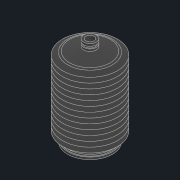
# Autodesk Inventor part: MCEN4000:T7
Saved by Autodesk Inventor 2021 (Build 250183000, 183)
## iProperties
Created: 2020-10-22
Part Number: MCEN4000:T7
Material: RUBBER, SILICONE
Document SubType Name: Modeling
Designer: Tang Kang Ning
Mass: 90.957 g
Surface Area: 1680.71 cm^2
Volume: 81.2116 cm^3
Density: 1.12 g/cm^3
Appearance: Rubber - Black
Description: BALL JOINT BELLOW
RevolveDIA: 7.056 mm
Author: Tang Kang Ning
Autodesk Inventor part; units mm, degrees
ref_plane "YZ Plane" through (0, 0, 0) normal (1, 0, 0) x (0, 1, 0)
ref_plane "XZ Plane" through (0, 0, 0) normal (0, 1, 0) x (-1, 0, 0)
ref_plane "XY Plane" through (0, 0, 0) normal (0, 0, 1) x (1, 0, 0)
sketch "Sketch1" plane through (0, 0, 0) normal (0, 0, 1) x (1, 0, 0)
  line L0 (-37, 65.25) -> (37, 65.25) projected
  line L1 (-37, 53.25) -> (37, 53.25) projected
  line L2 (35, 65.25) -> (35, 53.25)
  line L3 (7.056, 209) -> (7.056, 197)
  line L4 (7.056, 209) -> (7.056, 197)
  line L5 (9.056, 197) -> (7.056, 197)
  line L6 (7.056, 209) -> (11.056, 209)
  line L7 (35, 53.25) -> (39, 53.25)
  line L8 (39, 53.25) -> (39, 57.25)
  line L9 (39, 57.25) -> (37, 57.25)
  line L10 (37, 57.25) -> (37, 61.25)
  line L11 (37, 61.25) -> (39, 61.25)
  line L12 (39, 61.25) -> (39, 65.25)
  line L13 (39, 65.25) -> (37, 65.25) construction
  line L14 (11.056, 209) -> (11.056, 205)
  line L15 (11.056, 205) -> (9.056, 205)
  line L16 (9.056, 205) -> (9.056, 201)
  line L17 (9.056, 201) -> (11.056, 201)
  line L18 (11.056, 201) -> (11.056, 197)
  line L19 (39, 65.25) -> (47.9764, 69.6572)
  line L20 (37, 65.25) -> (45.9764, 69.6572)
  line L21 (37, 65.25) -> (37, 83.6946) construction
  line L22 (45.9764, 69.6572) -> (37, 69.6572) construction
  line L23 (45.9764, 69.6572) -> (37, 74.0645)
  line L24 (47.9764, 69.6572) -> (39, 74.0645)
  line L25 (35.5321, 190.0108) -> (11.056, 197.3225)
  line L26 (37, 188.6524) -> (9.056, 197)
  line L27 (37, 74.0645) -> (46.1526, 74.0645) construction
  line L28 (45.9764, 78.4717) -> (37, 82.8789)
  line L29 (47.9764, 78.4717) -> (39, 82.8789)
  line L30 (39, 74.0645) -> (47.9764, 78.4717)
  line L31 (37, 74.0645) -> (45.9764, 78.4717)
  line L32 (45.9764, 87.2861) -> (37, 91.6934)
  line L33 (47.9764, 87.2861) -> (39, 91.6934)
  line L34 (39, 82.8789) -> (47.9764, 87.2861)
  line L35 (37, 82.8789) -> (45.9764, 87.2861)
  line L36 (45.9764, 96.1006) -> (37, 100.5078)
  line L37 (47.9764, 96.1006) -> (39, 100.5078)
  line L38 (39, 91.6934) -> (47.9764, 96.1006)
  line L39 (37, 91.6934) -> (45.9764, 96.1006)
  line L40 (45.9764, 104.915) -> (37, 109.3223)
  line L41 (47.9764, 104.915) -> (39, 109.3223)
  line L42 (39, 100.5078) -> (47.9764, 104.915)
  line L43 (37, 100.5078) -> (45.9764, 104.915)
  line L44 (45.9764, 113.7295) -> (37, 118.1367)
  line L45 (47.9764, 113.7295) -> (39, 118.1367)
  line L46 (39, 109.3223) -> (47.9764, 113.7295)
  line L47 (37, 109.3223) -> (45.9764, 113.7295)
  line L48 (45.9764, 122.5439) -> (37, 126.9512)
  line L49 (47.9764, 122.5439) -> (39, 126.9512)
  line L50 (39, 118.1367) -> (47.9764, 122.5439)
  line L51 (37, 118.1367) -> (45.9764, 122.5439)
  line L52 (45.9764, 131.3584) -> (37, 135.7656)
  line L53 (47.9764, 131.3584) -> (39, 135.7656)
  line L54 (39, 126.9512) -> (47.9764, 131.3584)
  line L55 (37, 126.9512) -> (45.9764, 131.3584)
  line L56 (45.9764, 140.1729) -> (37, 144.5801)
  line L57 (47.9764, 140.1729) -> (39, 144.5801)
  line L58 (39, 135.7656) -> (47.9764, 140.1729)
  line L59 (37, 135.7656) -> (45.9764, 140.1729)
  line L60 (45.9764, 148.9873) -> (37, 153.3945)
  line L61 (47.9764, 148.9873) -> (39, 153.3945)
  line L62 (39, 144.5801) -> (47.9764, 148.9873)
  line L63 (37, 144.5801) -> (45.9764, 148.9873)
  line L64 (45.9764, 157.8018) -> (37, 162.209)
  line L65 (47.9764, 157.8018) -> (39, 162.209)
  line L66 (39, 153.3945) -> (47.9764, 157.8018)
  line L67 (37, 153.3945) -> (45.9764, 157.8018)
  line L68 (45.9764, 166.6162) -> (37, 171.0234)
  line L69 (47.9764, 166.6162) -> (39, 171.0234)
  line L70 (39, 162.209) -> (47.9764, 166.6162)
  line L71 (37, 162.209) -> (45.9764, 166.6162)
  line L72 (45.9764, 175.4307) -> (37, 179.8379)
  line L73 (47.9764, 175.4307) -> (39, 179.8379)
  line L74 (39, 171.0234) -> (47.9764, 175.4307)
  line L75 (37, 171.0234) -> (45.9764, 175.4307)
  line L76 (0, -41.8) -> (0, 250.8) projected
  line L77 (-9, 209) -> (9, 209) construction
  line L78 (45.9764, 184.2451) -> (37, 188.6524)
  line L79 (47.9764, 184.2451) -> (39, 188.6524)
  line L80 (39, 179.8379) -> (47.9764, 184.2451)
  line L81 (37, 179.8379) -> (45.9764, 184.2451)
  arc A0 (39, 188.6524) -> (35.5321, 190.0108) centre (29.1072, 168.5031) ccw
  point P0 (0, 0)
  point P1 (37, 195.25)
  dimension "d0" = 4
  dimension "d1" = 12
  dimension "d2" = 4
  dimension "d3" = 2
  dimension "d4" = 2
  dimension "d5" = 4
  dimension "d6" = 4
  dimension "d7" = 2
  dimension "d8" = 2
  dimension "d12" = 116.15
  dimension "d13" = 0.8814
  dimension "d17" = 10
  dimension "d18" = 8.8145
  dimension "d28" = 8.8145
  dimension "d34" = 12
  dimension "d35" = 4
  dimension "RevolveDIA" = 7.056
  dimension "d39" = 106.632
  dimension "d40" = 2
  dimension "d41" = 0.8814
  constraints: 155 end point, 10 perpendicular, 8 point on line, 4 horizontal, 4 vertical, 3 parallel, 2 point on circle, 2 tangent, 1 centre point, 1 coincident, 1 collinear, 1 equal length, 135 other
  measures "d0" distance between parallel lines of L13 L11
  measures "d1" distance of L2.start L2.end
  measures "d2" distance between parallel lines of L7 L9
  measures "d3" distance between parallel lines of L10 L12
  measures "d4" distance between parallel lines of L2 L10
  measures "d5" distance of L6.end L14.end
  measures "d6" distance of L17.end L18.end
  measures "d12" angle of L12 L19
  measures "d13" distance between parallel lines of L19 L20
  measures "d17" distance of L12.end L19.end
  measures "d18" distance of L0.end L23.end
  measures "d28" distance of L20.end L28.start
  measures "d34" distance of L3.start L3.end
  measures "d35" distance between parallel lines of L5 L17
  measures "RevolveDIA" distance between parallel lines of L3 L76
  measures "d39" angle of L25 L14
  measures "d40" distance of L5.start L3.end
  measures "d41" distance between parallel lines of L25 L26
revolve "Revolution1" add sketch "Sketch1" angle 360 about axis through (0, -10, 0) along (0, 1, 0) contours L0 L20 L23 L31 L28 L35 L32 L39 L36 L43 L40 L47 L44 L51 L48 L55 L52 L59 L56 L63 L60 L67 L64 L71 L68 L75 L72 L81 L78 L26 L5 L3 L6 L14 L15 L16 L17 L18 L25 A0 L79 L80 L73 L74 L69 L70 L65 L66 L61 L62 L57 L58 L53 L54 L49 L50 L45 L46 L41 L42 L37 L38 L33 L34 L29 L30 L24 L19 L12 L11 L10 L9 L8 L7 L1 L2
equation "\"d0\" = 0.333333 * d1"
equation "\"d2\" = d0"
equation "\"d5\" = d0"
equation "\"d6\" = d0"
equation "\"d28\" = d18"
equation "\"d40\" = d7"
equation "\"d41\" = d13"
equation "\"d10\" = d9"
equation "\"d9\" = 150.364378"
body "Solid1"
